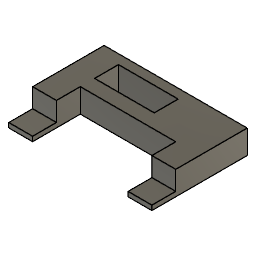
OLD Front Door Structure 25-03-2026 (Autodesk Fusion 360 design; units mm, degrees)
part number: 2026-03-10-09-19-59-139
Autodesk Fusion 360 part; units mm, degrees
sketch "Esquisse2" plane through (0, 0, 0) normal (0, 0, 1) x (1, 0, 0)
  line L0 (300, 0) -> (300, 200)
  line L1 (300, 200) -> (0, 200)
  line L2 (0, 200) -> (0, 0)
  line L3 (250, 0) -> (250, 100)
  line L4 (250, 100) -> (50, 100)
  line L5 (50, 100) -> (50, 0)
  line L6 (50, 180) -> (175, 180)
  line L7 (175, 180) -> (175, 130)
  line L8 (175, 130) -> (50, 130)
  line L9 (50, 130) -> (50, 180)
  line L10 (0, 0) -> (50, 0)
  line L11 (250, 0) -> (300, 0)
  dimension "d7" = 300
  dimension "d8" = 200
  dimension "d9" = 200
  dimension "d10" = 100
  dimension "d11" = 50
  dimension "d12" = 125
  dimension "d13" = 50
  constraint vertical L0
  constraint horizontal L1
  constraint vertical L2
  constraint coincident L2.end L10.start
  constraint vertical L3
  constraint horizontal L4
  constraint vertical L5
  constraint horizontal L6
  constraint vertical L7
  constraint horizontal L8
  constraint vertical L9
  constraint perpendicular L5 L10
  constraint perpendicular L0 L11
  measures "d7" distance of L2.end L0.start
  measures "d8" distance of L2.end L1.end
  measures "d9" distance of L5.end L3.start
  measures "d10" distance of L5.end L4.end
  measures "d11" distance of L2.end L5.end
  measures "d12" distance of L6.start L6.end
  measures "d13" distance of L6.start L8.end
extrude "Extrusion2" add sketch "Esquisse2" along normal blind 50
sketch "Esquisse3" plane through (300, 0, 0) normal (1, 0, 0) x (0, 1, 0)
  line L0 (0, 0) -> (200, 0)
  line L1 (200, 0) -> (200, 50)
  line L2 (200, 50) -> (0, 50)
  line L3 (0, 50) -> (0, 0)
  line L4 (0, 50) -> (50, 50)
  line L5 (50, 50) -> (50, 10)
  line L6 (50, 10) -> (0, 10)
  line L7 (0, 10) -> (0, 50)
  dimension "d16" = 50
  dimension "d17" = 40
  constraint horizontal L4
  constraint vertical L5
  constraint horizontal L6
  constraint vertical L7
  constraint coincident L2.end L3.start
  measures "d16" distance of L2.end L4.end
  measures "d17" distance of L2.end L6.end
extrude "Extrusion3" cut sketch "Esquisse3" against normal blind 300 contours L2 L3 L4 L5 L6 L7
